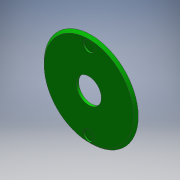
# Autodesk Inventor part: cuello
Saved by Autodesk Inventor 2016 (Build 200138000, 138)
## iProperties
Created: 2016-02-19
Part Number: cuello
Material: Genérico
Document SubType Name: Modeling
Designer: Usuario1
Density: 1 g/cm^3
Appearance: Valor por defecto
Author: Usuario1
Autodesk Inventor part; units mm, degrees
ref_plane "YZ Plane" through (0, 0, 0) normal (1, 0, 0) x (0, 1, 0)
ref_plane "XZ Plane" through (0, 0, 0) normal (0, 1, 0) x (-1, 0, 0)
ref_plane "XY Plane" through (0, 0, 0) normal (0, 0, 1) x (1, 0, 0)
sketch "Boceto1" plane through (0, 0, 0) normal (0, 0, 1) x (1, 0, 0)
  line L0 (2.7328, 4.3298) -> (8.5721, 4.3298)
  line L1 (3.0328, 4.0298) -> (8.5721, 4.0298)
  line L2 (8.5721, 4.3298) -> (8.5721, 4.0298)
  line L3 (2.7328, 4.3298) -> (3.0328, 4.0298)
  point P0 (0, 0)
  constraints: 8 end point
revolve "Revolución1" add sketch "Boceto1" angle 360 about axis through (8.5721, 4.3298, 0) along (0, -1, 0)
sketch "Boceto3" plane through (8.5721, 4.0298, 0) normal (0, -1, 0) x (1, 0, 0)
  circle A0 centre (0, 0) radius 5.5393 projected
  circle A1 centre (0, 0) radius 5.8393
  circle A2 centre (0, 4.7895) radius 0.675
  circle A3 centre (0, -4.7895) radius 0.675
  point P0 (-8.5721, 0)
  point P1 (0, -4.7895)
  dimension "d5" = 1.35
  dimension "d6" = 1.35
  constraints: 3 centre point
  measures "d5" diameter of A2
  measures "d6" diameter of A3
extrude "Extrusión2" cut sketch "Boceto3" against normal blind 0.17 contours A2 | A3
sketch "Boceto4" plane through (8.5721, 4.0298, 0) normal (0, -1, 0) x (1, 0, 0)
  circle A0 centre (0, 0) radius 5.5393 projected
  circle A1 centre (0, 0) radius 1.55
  point P0 (-8.5721, 0)
  dimension "d9" = 3.1
  constraints: 1 centre point, 1 coincident
  measures "d9" diameter of A1
extrude "Extrusión3" cut sketch "Boceto4" against normal blind 10 contours A1
